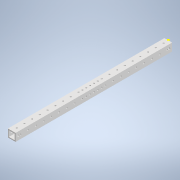
# Autodesk Inventor part: 1x1x20.25
Saved by Autodesk Inventor 2020 (Build 240168000, 168)
## iProperties
Created: 2020-01-19
Part Number: 1x1x20.25
Material: Generic
Document SubType Name: Modeling
Designer: srini
Density: 1 g/cm^3
Appearance: Default
Author: srini
Autodesk Inventor part; units mm, degrees
ref_plane "YZ Plane" through (0, 0, 0) normal (1, 0, 0) x (0, 1, 0)
ref_plane "XZ Plane" through (0, 0, 0) normal (0, 1, 0) x (-1, 0, 0)
ref_plane "XY Plane" through (0, 0, 0) normal (0, 0, 1) x (1, 0, 0)
sketch "Sketch1" plane through (0, 0, 0) normal (0, 0, 1) x (1, 0, 0)
  line L0 (-12.7, -12.7) -> (12.7, -12.7)
  line L1 (12.7, -12.7) -> (12.7, 12.7)
  line L2 (12.7, 12.7) -> (-12.7, 12.7)
  line L3 (-12.7, 12.7) -> (-12.7, -12.7)
  line L4 (-12.7, -12.7) -> (12.7, 12.7) construction
  line L5 (12.7, -12.7) -> (-12.7, 12.7) construction
  line L6 (-9.525, 9.525) -> (9.525, 9.525)
  line L7 (9.525, 9.525) -> (9.525, -9.525)
  line L8 (9.525, -9.525) -> (-9.525, -9.525)
  line L9 (-9.525, -9.525) -> (-9.525, 9.525)
  point P0 (0, 0)
  dimension "d0" = 25.4
  dimension "d1" = 25.4
  dimension "d2" = 3.175
  constraints: 20 end point, 4 parallel, 2 midpoint, 2 perpendicular, 1 horizontal, 3 other
  measures "d0" distance of L1.end L2.end
  measures "d1" distance of L0.end L1.end
  measures "d2" distance between parallel lines of L6 L2
extrude "Extrusion1" add sketch "Sketch1" along normal blind 514.35
sketch "Sketch2" plane through (-12.7, 12.7, 0) normal (0, 1, 0) x (1, 0, 0)
  circle A0 centre (12.7, -15.875) radius 2.54
  line L0 (0, 0) -> (0, -514.35) projected
  line L1 (25.4, 0) -> (0, 0) projected
  circle A1 centre (12.7, -41.275) radius 2.54
  circle A2 centre (12.7, -66.675) radius 2.54
  circle A3 centre (12.7, -92.075) radius 2.54
  circle A4 centre (12.7, -117.475) radius 2.54
  circle A5 centre (12.7, -142.875) radius 2.54
  circle A6 centre (12.7, -168.275) radius 2.54
  circle A7 centre (12.7, -193.675) radius 2.54
  circle A8 centre (12.7, -219.075) radius 2.54
  circle A9 centre (12.7, -244.475) radius 2.54
  circle A10 centre (12.7, -269.875) radius 2.54
  circle A11 centre (12.7, -295.275) radius 2.54
  circle A12 centre (12.7, -320.675) radius 2.54
  circle A13 centre (12.7, -346.075) radius 2.54
  circle A14 centre (12.7, -371.475) radius 2.54
  circle A15 centre (12.7, -396.875) radius 2.54
  circle A16 centre (12.7, -422.275) radius 2.54
  circle A17 centre (12.7, -447.675) radius 2.54
  circle A18 centre (12.7, -473.075) radius 2.54
  circle A19 centre (12.7, -498.475) radius 2.54
  point P0 (12.7, 0)
  dimension "d5" = 12.7
  dimension "d6" = 15.875
  dimension "d7" = 5.08
  dimension "d10" = 25.4
  constraints: 20 centre point, 1 vertical, 38 other
  measures "d5" distance from line of A0.centre L0
  measures "d6" distance from line of A0.centre L1
  measures "d7" diameter of A0
  measures "d10" distance of A0.centre A1.centre
extrude "Extrusion2" cut sketch "Sketch2" against normal through all
sketch "Sketch3" plane through (12.7, -12.7, 0) normal (1, 0, 0) x (0, 0, -1)
  circle A0 centre (-15.875, 12.7) radius 2.54
  line L0 (0, 0) -> (-514.35, 0) projected
  line L1 (0, 0) -> (0, 25.4) projected
  circle A1 centre (-41.275, 12.7) radius 2.54
  circle A2 centre (-66.675, 12.7) radius 2.54
  circle A3 centre (-92.075, 12.7) radius 2.54
  circle A4 centre (-117.475, 12.7) radius 2.54
  circle A5 centre (-142.875, 12.7) radius 2.54
  circle A6 centre (-168.275, 12.7) radius 2.54
  circle A7 centre (-193.675, 12.7) radius 2.54
  circle A8 centre (-219.075, 12.7) radius 2.54
  circle A9 centre (-244.475, 12.7) radius 2.54
  circle A10 centre (-269.875, 12.7) radius 2.54
  circle A11 centre (-295.275, 12.7) radius 2.54
  circle A12 centre (-320.675, 12.7) radius 2.54
  circle A13 centre (-346.075, 12.7) radius 2.54
  circle A14 centre (-371.475, 12.7) radius 2.54
  circle A15 centre (-396.875, 12.7) radius 2.54
  circle A16 centre (-422.275, 12.7) radius 2.54
  circle A17 centre (-447.675, 12.7) radius 2.54
  circle A18 centre (-473.075, 12.7) radius 2.54
  circle A19 centre (-498.475, 12.7) radius 2.54
  point P0 (0, 12.7)
  dimension "d17" = 12.7
  dimension "d18" = 15.875
  dimension "d19" = 5.08
  dimension "d22" = 25.4
  constraints: 20 centre point, 1 horizontal, 38 other
  measures "d17" distance from line of A0.centre L0
  measures "d18" distance from line of A0.centre L1
  measures "d19" diameter of A0
  measures "d22" distance of A0.centre A1.centre
extrude "Extrusion3" cut sketch "Sketch3" against normal through all
sketch "Sketch4" plane through (-12.7, 12.7, 0) normal (0, 1, 0) x (1, 0, 0)
  point P0 (12.7, 0)
sketch "Sketch5" plane through (12.7, -12.7, 0) normal (1, 0, 0) x (0, 0, -1)
  circle A0 centre (-9.525, 12.7) radius 3.3528 projected
  circle A1 centre (-504.825, 12.7) radius 3.3528 projected
  point P0 (0, 12.7)
extrude "Extrusion4" cut sketch "Sketch5" against normal through all
sketch "Sketch6" plane through (12.7, -12.7, 0) normal (1, 0, 0) x (0, 0, -1)
  circle A0 centre (-282.575, 12.7) radius 2.54
  line L0 (-257.175, -26.6173) -> (-257.175, 80.6593) construction
  line L1 (-514.35, 0) -> (-514.35, 25.4) projected
  circle A1 centre (-320.675, 12.7) radius 2.54 construction
  line L2 (0, 25.4) -> (-514.35, 25.4) projected
  circle A2 centre (-257.175, 12.7) radius 2.54
  circle A3 centre (-231.775, 12.7) radius 2.54
  point P0 (0, 12.7)
  dimension "d31" = 257.175
  dimension "d32" = 38.1
  dimension "d35" = 25.4
  constraints: 3 centre point, 2 end point, 1 equal radius, 1 horizontal, 1 horizontal alignment, 1 vertical, 4 other
  measures "d31" distance between parallel lines of L0 L1
  measures "d32" distance of A1.centre A0.centre
  measures "d35" distance of A0.centre A2.centre
extrude "Extrusion5" cut sketch "Sketch6" against normal through all
sketch "Sketch8" plane through (-12.7, 12.7, 0) normal (0, 1, 0) x (1, 0, 0)
  circle A0 centre (12.7, -231.775) radius 2.54
  line L0 (0, 0) -> (0, -514.35) projected
  circle A1 centre (12.7, -219.075) radius 2.54 construction
  circle A2 centre (12.7, -257.175) radius 2.54
  circle A3 centre (12.7, -282.575) radius 2.54
  point P0 (12.7, 0)
  dimension "d42" = 12.7
  dimension "d45" = 25.4
  constraints: 3 centre point, 1 equal radius, 1 vertical, 1 vertical alignment, 4 other
  measures "d42" distance of A0.centre A1.centre
  measures "d45" distance of A0.centre A2.centre
extrude "Extrusion6" cut sketch "Sketch8" against normal through all
body "Solid1"
